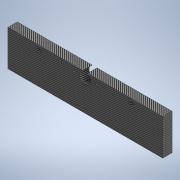
# Autodesk Inventor part: 006
Saved by Autodesk Inventor 2022.2 (Build 262287000, 287)
## iProperties
Manager: Angie Guevara
Company: ITM
Created: 2021-11-08
Part Number: 006
Material: CFRP
Document SubType Name: Modeling
Designer: Samuel Gómez
Density: 1.43 g/cm^3
Appearance: Carbon Fiber
Checked By: Angie Guevara
Engr Approved By: Angie Guevara
Engineer: Angie Guevara
Author: Samuel Gómez
Autodesk Inventor part; units mm, degrees
ref_plane "YZ Plane" through (0, 0, 0) normal (1, 0, 0) x (0, 1, 0)
ref_plane "XZ Plane" through (0, 0, 0) normal (0, 1, 0) x (-1, 0, 0)
ref_plane "XY Plane" through (0, 0, 0) normal (0, 0, 1) x (1, 0, 0)
sketch "Boceto1" plane through (0, 0, 0) normal (0, 0, 1) x (1, 0, 0)
  line L0 (0, 0) -> (300, 0)
  line L1 (300, 0) -> (300, -70)
  line L2 (300, -70) -> (0, -70)
  line L3 (0, -70) -> (0, 0)
  dimension "d0" = 300
  dimension "d1" = 70
  constraints: 8 end point, 2 parallel, 1 horizontal, 1 perpendicular
  measures "d0" distance of L0.start L0.end
  measures "d1" distance of L0.end L1.end
extrude "Extrusión1" add sketch "Boceto1" along normal blind 18
sketch "Boceto2" plane through (0, 0, 18) normal (0, 0, 1) x (1, 0, 0)
  line L0 (300, 0) -> (0, 0) construction
  line L1 (150, 0) -> (150, -70) construction
  line L2 (0, -70) -> (300, -70) construction
  line L3 (0, 0) -> (0, -70) construction
  line L4 (0, -35) -> (300, -35) construction
  line L5 (300, -70) -> (300, 0) construction
  circle A0 centre (150, -10) radius 11
  line L6 (145.4175, 0) -> (154.5825, 0) construction
  line L7 (150, -10) -> (113.1437, -10) construction
  circle A1 centre (128.0797, -10) radius 1.5
  line L8 (150, -10) -> (186.8563, -10) construction
  circle A2 centre (171.9203, -10) radius 1.5
  circle A3 centre (150, -31.9203) radius 1.5
  line L9 (150, -10) -> (125.2951, -34.7049)
  line L10 (150, -10) -> (165.139, -25.139)
  dimension "d4" = 22
  dimension "d5" = 4.5825
  dimension "d6" = 3
  dimension "d8" = 3
  dimension "d17" = 45
  dimension "d18" = 45
  dimension "d20" = 15.5
  dimension "d22" = 15.5
  constraints: 14 end point, 6 midpoint, 4 centre point, 4 point on line, 2 horizontal, 2 point on circle, 2 symmetric about line, 1 other
  measures "d4" diameter of A0
  measures "d5" distance from line of L6.start L1
  measures "d6" diameter of A1
  measures "d8" diameter of A3
  measures "d17" angle of L1 L9
  measures "d18" angle of L1 L10
  measures "d20" distance from line of L10 A2.centre
  measures "d22" distance from line of L10 A3.centre
extrude "Extrusión2" cut sketch "Boceto2" against normal blind 18
sketch "Boceto3" plane through (0, 0, 18) normal (0, 0, 1) x (1, 0, 0)
  circle A0 centre (240, -8.01) radius 4
  arc A1 (145.4175, 0) -> (154.5825, 0) centre (150, -10) ccw projected
  line L0 (150, -10) -> (150, 29.6018) construction
  circle A2 centre (60, -8.01) radius 4
  point P0 (0, 0)
  dimension "d12" = 8
  dimension "d13" = 90
  dimension "d14" = 1.99
  constraints: 2 centre point, 2 end point, 1 symmetric about line, 1 vertical, 1 other
  measures "d12" diameter of A0
  measures "d13" horizontal distance of A0.centre L0.start
  measures "d14" vertical distance of L0.start A0.centre
extrude "Extrusión3" cut sketch "Boceto3" against normal blind 18
